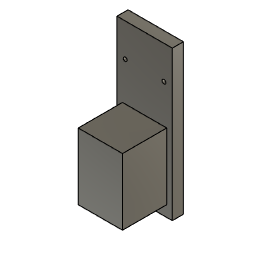
Laser Head v2 (Autodesk Fusion 360 design; units mm, degrees)
Autodesk Fusion 360 part; units mm, degrees
sketch "Sketch1" plane through (0, 0, 0) normal (0, 0, 1) x (1, 0, 0)
  line L0 (0, 40) -> (40, 40)
  line L1 (40, 40) -> (40, 0)
  line L2 (40, 0) -> (0, 0)
  line L3 (0, 0) -> (0, 40)
  line L4 (-5, 50) -> (45, 50)
  line L5 (45, 50) -> (45, 40)
  line L6 (45, 40) -> (-5, 40)
  line L7 (-5, 40) -> (-5, 50)
  dimension "d1" = 40
  dimension "d2" = 40
  dimension "d3" = 40
  dimension "d4" = 40
  dimension "d5" = 45
  dimension "d6" = 50
  dimension "d7" = 50
  dimension "d8" = 10
  constraint horizontal L0
  constraint vertical L1
  constraint horizontal L2
  constraint vertical L3
  constraint horizontal L4
  constraint vertical L5
  constraint horizontal L6
  constraint vertical L7
  measures "d1" distance of L2.end L0
  measures "d2" distance of L2.end L1
  measures "d3" distance of L0.end L1.end
  measures "d4" distance of L0.start L0.end
  measures "d5" distance of L2.end L5
  measures "d6" distance of L4.start L4.end
  measures "d7" distance of L2.end L4
  measures "d8" distance of L4.start L6.end
extrude "Extrude1" add sketch "Sketch1" along normal blind 60 contours L0 L1 L2 L3 L6 makes body 1
extrude "Extrude2" add sketch "Sketch1" along normal blind 135 separate body contours L0 L4 L5 L6 L7 makes body 2
move_body "Move1" bodies 1 to x (1, 0, 0) y (0, 1, 0) z (0, 0, 1) at (0, 0, 10)
sketch "Sketch2" plane through (0, 50, 0) normal (0, 1, 0) x (-1, 0, 0)
  line L0 (-45, 0) -> (5, 0)
  line L1 (5, 0) -> (5, 135)
  line L2 (5, 135) -> (-45, 135)
  line L3 (-45, 135) -> (-45, 0)
  circle A0 centre (-2.5, 30) radius 1.75
  circle A1 centre (-37.5, 30) radius 1.75
  circle A2 centre (-2.5, 105) radius 1.75
  circle A3 centre (-37.5, 105) radius 1.75
  dimension "d13" = 5
  dimension "d14" = 3.5
  dimension "d15" = 2.5
  dimension "d16" = 30
  dimension "d19" = -35
  dimension "d20" = 75
  measures "d13" distance of origin L0.end
  measures "d14" diameter of A0
  measures "d15" horizontal distance of origin A0.centre
  measures "d16" vertical distance of origin A0.centre
extrude "Extrude3" cut sketch "Sketch2" against normal blind 35 contours A0 | A1 | A2 | A3 bodies 1 2
